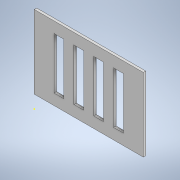
# Autodesk Inventor part: frount plate
Saved by Autodesk Inventor 2021 (Build 250183000, 183)
## iProperties
Created: 2021-07-05
Part Number: frount plate
Material: Generic
Document SubType Name: Modeling
Designer: newic
Density: 1 g/cm^3
Appearance: Default
Author: newic
Autodesk Inventor part; units mm, degrees
ref_plane "YZ Plane" through (0, 0, 0) normal (1, 0, 0) x (0, 1, 0)
ref_plane "XZ Plane" through (0, 0, 0) normal (0, 1, 0) x (-1, 0, 0)
ref_plane "XY Plane" through (0, 0, 0) normal (0, 0, 1) x (1, 0, 0)
sketch "Sketch1" plane through (0, 0, 0) normal (0, 0, 1) x (1, 0, 0)
  line L0 (0, 0) -> (139.7, 0)
  line L1 (139.7, 0) -> (139.7, 127)
  line L2 (139.7, 127) -> (0, 127)
  line L3 (0, 127) -> (0, 0)
  dimension "d0" = 139.7
  dimension "d1" = 127
  constraints: 8 end point, 2 parallel, 1 horizontal, 1 perpendicular
  measures "d0" distance of L2.end L1.end
  measures "d1" distance of L1.end L0.end
extrude "Extrusion1" add sketch "Sketch1" along normal blind 3.175
sketch "Sketch2" plane through (0, 0, 3.175) normal (0, 0, 1) x (1, 0, 0)
  line L0 (0, 0) -> (139.7, 0) projected
  line L1 (139.7, 0) -> (139.7, 127) projected
  line L2 (0, 0) -> (139.7, 0)
  line L3 (139.7, 0) -> (139.7, 19.05)
  line L4 (139.7, 19.05) -> (0, 19.05)
  line L5 (0, 19.05) -> (0, 0)
  line L6 (139.7, 127) -> (0, 127) projected
  line L7 (0, 127) -> (19.05, 127)
  line L8 (0, 86.1969) -> (0, 127)
  line L9 (0, 127) -> (139.7, 127)
  line L10 (139.7, 127) -> (139.7, 107.95)
  line L11 (139.7, 107.95) -> (0, 107.95)
  line L12 (0, 107.95) -> (0, 127)
  line L13 (0, 127) -> (19.05, 127)
  line L14 (19.05, 127) -> (19.05, 0)
  line L15 (19.05, 0) -> (0, 0)
  line L16 (0, 0) -> (0, 127)
  line L17 (139.7, 0) -> (120.65, 0)
  line L18 (120.65, 0) -> (120.65, 127)
  line L19 (120.65, 127) -> (139.7, 127)
  line L20 (139.7, 127) -> (139.7, 0)
  point P0 (19.05, 19.05)
  point P1 (19.05, 107.95)
  point P2 (120.65, 107.95)
  point P3 (120.65, 19.05)
  dimension "d4" = 19.05
  dimension "d6" = 19.05
  dimension "d7" = 19.05
  constraints: 36 end point, 8 parallel, 5 horizontal, 4 perpendicular, 4 point on line
  measures "d4" distance of L3.end L2.end
  measures "d6" distance of L9.end L10.end
  measures "d7" distance of L18.end L19.end
extrude "Extrusion2" add sketch "Sketch2" along normal blind 3.175 contours L5 L4 L14 L0 | L14 L4 L18 L0 | L16 L8 L11 L14 L4 | L18 L4 L1 L0 | L18 L11 L1 L4 | L14 L6 L18 L11 | L11 L8 L6 L14 | L18 L6 L1 L11
sketch "Sketch3" plane through (0, 0, 0) normal (0, 0, -1) x (-1, 0, 0)
  line L0 (-19.05, 19.05) -> (-120.65, 19.05) projected
  line L1 (-120.65, 107.95) -> (-19.05, 107.95) projected
  line L2 (-25.4, 107.95) -> (-25.4, 19.05)
  line L3 (-19.05, 107.95) -> (-19.05, 19.05) projected
  line L4 (-38.1, 107.95) -> (-38.1, 19.05)
  line L5 (-114.3, 107.95) -> (-114.3, 19.05)
  line L6 (-101.6, 107.95) -> (-101.6, 19.05)
  line L7 (-120.65, 19.05) -> (-120.65, 107.95) projected
  line L8 (-88.9, 107.95) -> (-88.9, 19.05)
  line L9 (-50.8, 107.95) -> (-50.8, 19.05)
  line L10 (-76.2, 107.95) -> (-76.2, 19.05)
  line L11 (-63.5, 107.95) -> (-63.5, 19.05)
  line L12 (-130.7408, 107.95) -> (-4.1346, 107.95)
  line L13 (0, 127) -> (0, 0) projected
  line L14 (-128.9627, 19.05) -> (-12.6698, 19.05)
  line L15 (-128.9627, 30.48) -> (-12.6698, 30.48)
  line L16 (-130.7408, 96.52) -> (-4.1346, 96.52)
  point P0 (-25.4, 96.52)
  point P1 (-38.1, 96.52)
  point P2 (-38.1, 30.48)
  point P3 (-25.4, 30.48)
  point P4 (-50.8, 96.52)
  point P5 (-63.5, 96.52)
  point P6 (-63.5, 30.48)
  point P7 (-50.8, 30.48)
  point P8 (-76.2, 96.52)
  point P9 (-88.9, 96.52)
  point P10 (-88.9, 30.48)
  point P11 (-76.2, 30.48)
  point P12 (-101.6, 96.52)
  point P13 (-114.3, 96.52)
  point P14 (-114.3, 30.48)
  point P15 (-101.6, 30.48)
  dimension "d14" = 12.7
  dimension "d15" = 6.35
  dimension "d17" = 12.7
  dimension "d18" = 12.7
  dimension "d19" = 12.7
  dimension "d20" = 12.7
  dimension "d21" = 12.7
  dimension "d22" = 12.7
  dimension "d23" = 11.43
  dimension "d24" = 11.43
  constraints: 24 end point, 8 parallel, 4 point on line, 1 horizontal, 1 perpendicular
  measures "d14" distance between parallel lines of L2 L4
  measures "d15" distance between parallel lines of L3 L2
  measures "d17" distance between parallel lines of L5 L6
  measures "d18" distance between parallel lines of L6 L8
  measures "d19" distance between parallel lines of L4 L9
  measures "d20" distance between parallel lines of L8 L10
  measures "d21" distance between parallel lines of L9 L11
  measures "d22" distance between parallel lines of L11 L10
  measures "d23" distance between parallel lines of L14 L15
  measures "d24" distance between parallel lines of L12 L16
extrude "Extrusion3" cut sketch "Sketch3" against normal through all contours L15 L4 L16 L2 | L15 L11 L16 L9 | L15 L8 L16 L10 | L15 L5 L16 L6
sketch "Sketch4" plane through (0, 0, 0) normal (0, 0, -1) x (-1, 0, 0)
  line L0 (-120.65, 19.05) -> (-120.65, 107.95) projected
  line L1 (-120.65, 107.95) -> (-19.05, 107.95) projected
  line L2 (-19.05, 107.95) -> (-19.05, 19.05) projected
  line L3 (-19.05, 19.05) -> (-120.65, 19.05) projected
  line L4 (-139.7, 127) -> (0, 127) projected
  line L5 (0, 0) -> (-139.7, 0) projected
  line L6 (-157.0502, 127) -> (65.2705, 127)
  line L7 (-157.0502, 110.49) -> (65.2705, 110.49)
  line L8 (-152.5949, 0) -> (41.6573, 0)
  line L9 (-152.5949, 16.51) -> (41.6573, 16.51)
  line L10 (-147.9168, 24.0704) -> (-145.2436, -7.3397)
  line L11 (8.7478, 21.5847) -> (14.9253, -14.4682)
  line L12 (-146.5802, 130.3299) -> (-146.5802, 103.3752)
  line L13 (-146.5802, 103.3752) -> (-146.5802, 100.0337)
  line L14 (14.9253, 133.2259) -> (10.47, 95.1328)
  point P0 (12.4462, 0)
  point P1 (9.6173, 16.51)
  point P2 (-147.2734, 16.51)
  point P3 (-145.8683, 0)
  point P4 (12.2662, 110.49)
  point P5 (14.1972, 127)
  point P6 (0, 127)
  point P7 (-146.5802, 127)
  point P8 (-146.5802, 110.49)
  dimension "d27" = 127
  dimension "d28" = 16.51
  dimension "d29" = 16.51
  constraints: 18 end point, 2 horizontal, 2 parallel, 1 point on line, 1 vertical
  measures "d27" distance between parallel lines of L4 L5
  measures "d28" distance between parallel lines of L6 L7
  measures "d29" distance between parallel lines of L8 L9
extrude "Extrusion4" cut sketch "Sketch4" against normal through all contours L4 L6 L14 L7 L12 | L5 L8 L10 L9 L11
sketch "Sketch6" plane through (139.7, 16.51, 0) normal (1, 0, 0) x (0, 0, -1)
  line L0 (-6.35, 0) -> (-6.35, 93.98) projected
  line L1 (-6.35, 93.98) -> (-3.175, 93.98)
  line L2 (-3.175, 93.98) -> (-3.175, -1176.02)
  line L3 (-3.175, -1176.02) -> (-6.35, -1176.02)
  line L4 (-6.35, -1176.02) -> (-6.35, 93.98)
  point P0 (0, -16.51)
  dimension "d32" = 3.175
  dimension "d33" = 1270
  constraints: 8 end point, 2 parallel, 1 horizontal, 1 perpendicular
  measures "d32" distance of L2.end L3.end
  measures "d33" distance of L1.end L2.end
extrude "Extrusion5" cut sketch "Sketch6" against normal through all
sketch "Sketch7" plane through (0, 0, 3.175) normal (0, 0, 1) x (1, 0, 0)
  point P0 (0, 0)
body "Solid1"
